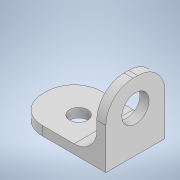
# Autodesk Inventor part: prependicular
Saved by Autodesk Inventor 2020 (Build 240168000, 168)
## iProperties
Created: 2019-06-20
Part Number: prependicular
Material: Generic
Document SubType Name: Modeling
Designer: Vivek Muskan
Density: 1 g/cm^3
Appearance: Default
Author: Vivek Muskan
Autodesk Inventor part; units mm, degrees
ref_plane "YZ Plane" through (0, 0, 0) normal (1, 0, 0) x (0, 1, 0)
ref_plane "XZ Plane" through (0, 0, 0) normal (0, 1, 0) x (-1, 0, 0)
ref_plane "XY Plane" through (0, 0, 0) normal (0, 0, 1) x (1, 0, 0)
sketch "Sketch1" plane through (0, 0, 0) normal (0, 0, 1) x (1, 0, 0)
  line L0 (0, 0) -> (-20, 0)
  line L1 (-20, 0) -> (-20, 2)
  line L2 (-20, 2) -> (0, 2)
  line L3 (0, 2) -> (0, 0)
  line L4 (0, 0) -> (-2, 0)
  line L5 (-2, 0) -> (-2, 15)
  line L6 (-2, 15) -> (0, 15)
  line L7 (0, 15) -> (0, 0)
  point P0 (-2, 2)
  dimension "d0" = 20
  dimension "d1" = 2
  dimension "d2" = 2
  dimension "d3" = 15
  constraints: 16 end point, 4 parallel, 2 horizontal, 2 perpendicular
  measures "d0" distance of L1.end L2.end
  measures "d1" distance of L0.end L1.end
  measures "d2" distance of L5.end L6.end
  measures "d3" distance of L4.end L5.end
extrude "Extrusion1" add sketch "Sketch1" along normal blind 13
fillet "Fillet1" radius 5 1 edges at (-2, 2, 6.5)
fillet "Fillet2" radius 6 4 edges at (-1, 15, 13) (-1, 15, 0) (-20, 1, 13) (-20, 1, 0)
sketch "Sketch2" plane through (0, 0, 13) normal (1, 0, 0) x (0, 0, -1)
  line L0 (13, 0) -> (0, 0) projected
  line L1 (6.5, 0) -> (6.5, 9)
  circle A0 centre (6.5, 9) radius 3
  dimension "d8" = 9
  dimension "d9" = 6
  constraints: 2 end point, 1 centre point, 1 coincident, 1 midpoint, 1 vertical
  measures "d8" distance of L1.start L1.end
  measures "d9" diameter of A0
extrude "Extrusion2" cut sketch "Sketch2" against normal blind 13
sketch "Sketch3" plane through (0, 0, 0) normal (0, -1, 0) x (1, 0, 0)
  line L0 (0, 7) -> (-2, 7) projected
  line L1 (0, 7) -> (-12, 7)
  circle A0 centre (-12, 7) radius 2
  point P0 (0, 0)
  dimension "d12" = 12
  dimension "d13" = 4
  constraints: 2 end point, 1 centre point, 1 coincident, 1 horizontal
  measures "d12" distance of L0.start L1.end
  measures "d13" diameter of A0
extrude "Extrusion3" cut sketch "Sketch3" against normal blind 13
body "Solid1"
